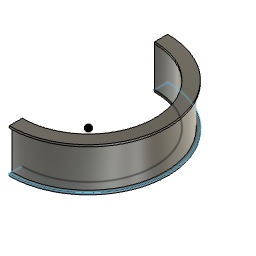
FC-50BandAdapter v2 (Autodesk Fusion 360 design; units mm, degrees)
Autodesk Fusion 360 part; units mm, degrees
note: some values were not read from the file. Set by a fixed rule: which sketch regions a step uses.
sketch "スケッチ1" plane through (0, 0, 0) normal (0, 0, 1) x (1, 0, 0)
  circle A0 centre (0, 0) radius 34.25
  circle A1 centre (0, 0) radius 39.5
  line L0 (0, 0) -> (0, 39.5)
  line L1 (0, 0) -> (0, -39.5)
  dimension "d1" = 68.5
  dimension "d2" = 79
  constraint coincident A0.centre A1.centre
  constraint concentric A0 A1
  constraint coincident A1 L0.end
  constraint vertical L0
  constraint coincident A1 L1.end
  constraint parallel L0 L1
  measures "d1" diameter of A0
  measures "d2" diameter of A1
extrude "押し出し1" add sketch "スケッチ1" along normal blind 20.5 contours A0 A1 L0 L1 picked at (1.8738, 37.616) makes body 1
sketch "スケッチ2" plane through (0, 0, 0) normal (0, 1, 0) x (1, 0, 0)
sketch "スケッチ3" plane through (0, 0, 0) normal (0, 0, 1) x (1, 0, 0)
  arc A0 (0, -41) -> (0, 41) centre (0, 0) ccw
  arc A1 (0, -34.25) -> (0, 34.25) centre (0, 0) ccw
  line L0 (0, 41) -> (0, 34.25)
  line L1 (0, -34.25) -> (0, -41)
  dimension "d8" = 34.25
  constraint coincident A0.centre A1.centre
  constraint vertical L0
  constraint parallel L0 L1
  measures "d8" radius of A1
sketch "スケッチ4" plane through (0, 0, 0) normal (0, 0, 1) x (1, 0, 0)
sketch "スケッチ5" plane through (0, 0, 0) normal (0, 0, 1) x (1, 0, 0)
extrude "押し出し2" add sketch "スケッチ3" against normal blind 1 separate body makes body 2
extrude "押し出し3" add sketch "スケッチ3" along normal blind 1 separate body makes body 3
move_body "移動1" bodies 3 to x (1, 0, 0) y (0, 1, 0) z (0, 0, 1) at (0, 0, 20.5)
